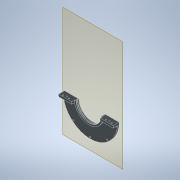
# Autodesk Inventor part: Крышка стенки картера низ
Saved by Autodesk Inventor 2021 (Build 250183000, 183)
## iProperties
Created: 2020-12-05
Part Number: Крышка стенки картера низ
Material: Чугун, серый
Document SubType Name: Modeling
Designer: Тимоха
Density: 7.15 g/cm^3
Appearance: Чугун серый
Mass: 3617.17 g
Surface Area: 1231.32 cm^2
Volume: 505.898 cm^3
Author: Тимоха
Autodesk Inventor part; units mm, degrees
ref_plane "YZ Plane" through (0, 0, 0) normal (1, 0, 0) x (0, 1, 0)
ref_plane "XZ Plane" through (0, 0, 0) normal (0, 1, 0) x (-1, 0, 0)
ref_plane "XY Plane" through (0, 0, 0) normal (0, 0, 1) x (1, 0, 0)
ref_plane "РабПлоскость1" through (7.7596, 35.7122, 0) normal (0, 0, 1) x (1, 0, 0)
sketch "Эскиз1" plane through (7.7596, 35.7122, 0) normal (0, 0, 1) x (1, 0, 0)
  circle A0 centre (-7.7596, -110.7122) radius 100 projected
  line L0 (177.2404, -110.7122) -> (177.2404, 289.2878) projected
  line L1 (157.2404, 304.2878) -> (157.2404, -110.7122) projected
  arc A1 (-172.7596, -110.7122) -> (157.2404, -110.7122) centre (-7.7596, -110.7122) ccw projected
  line L2 (-172.7596, -110.7122) -> (-172.7596, 304.2878) projected
  line L3 (-192.7596, 289.2878) -> (-192.7596, -110.7122) projected
  arc A2 (-192.7596, -110.7122) -> (177.2404, -110.7122) centre (-7.7596, -110.7122) ccw projected
  line L4 (-192.7596, -110.7122) -> (177.2404, -110.7122)
  circle A3 centre (-7.7596, -110.7122) radius 86
  line L5 (177.2404, 289.2878) -> (222.2404, 289.2878) projected
  line L6 (222.2404, 289.2878) -> (222.2404, 304.2878) projected
  line L7 (222.2404, 304.2878) -> (157.2404, 304.2878) projected
  line L8 (-172.7596, 304.2878) -> (-237.7596, 304.2878) projected
  line L9 (-237.7596, 304.2878) -> (-237.7596, 289.2878) projected
  line L10 (-237.7596, 289.2878) -> (-192.7596, 289.2878) projected
  point P0 (-7.7596, -35.7122)
  point P1 (177.2404, 304.2878)
  point P2 (-192.7596, 304.2878)
  point P3 (157.2404, -110.7122)
  point P4 (78.2404, -110.7122)
  point P5 (-93.7596, -110.7122)
  point P6 (-172.7596, -110.7122)
  dimension "d2" = 172
  constraints: 2 end point, 2 point on line, 1 centre point, 1 coincident, 1 perpendicular
  measures "d2" diameter of A3
extrude "Выдавливание1" add sketch "Эскиз1" along normal blind 10 contours L4 A1 A0 | A0 L4 A3 | L4 A2 A1 picked at (-5.6173, -205.81)
sketch "Эскиз2" plane through (7.7596, 35.7122, 10) normal (0, 0, 1) x (1, 0, 0)
  arc A0 (-93.7596, -110.7122) -> (78.2404, -110.7122) centre (-7.7596, -110.7122) ccw projected
  line L0 (-93.7596, -110.7122) -> (78.2404, -110.7122) projected
  line L1 (-93.7596, -110.7122) -> (78.2404, -110.7122) projected
  circle A1 centre (-7.7596, -110.7122) radius 97.5
  line L2 (-93.7596, -110.7122) -> (-105.2596, -110.7122)
  line L3 (78.2404, -110.7122) -> (89.7404, -110.7122)
  point P0 (-7.7596, -35.7122)
  point P1 (-172.7596, -110.7122)
  point P2 (157.2404, -110.7122)
  point P3 (-105.2596, -110.7122)
  point P4 (89.7404, -110.7122)
  point P5 (177.2404, -110.7122)
  dimension "d3" = 195
  constraints: 4 end point, 2 point on circle, 1 centre point, 1 coincident, 1 point on line
  measures "d3" diameter of A1
extrude "Выдавливание2" add sketch "Эскиз2" along normal blind 10 contours A0 L3 A1 L2
sketch "Эскиз3" plane through (0, 0, 0) normal (1, 0, 0) x (0, 1, 0)
  line L0 (-161, 20) -> (-75, 20) projected
  line L1 (-161, 20) -> (-161, 17)
  line L2 (-161, 20) -> (-161, 0) projected
  line L3 (-161, 17) -> (-168, 17)
  line L4 (-168, 17) -> (-168, 12)
  line L5 (-168, 12) -> (-161, 12)
  line L6 (-161, 12) -> (-161, 9)
  line L7 (-161, 9) -> (-168, 9)
  line L8 (-168, 9) -> (-168, 3)
  line L9 (-168, 3) -> (-161, 3)
  line L10 (-161, 0) -> (-75, 0) projected
  line L11 (-161, 3) -> (-161, 0)
  line L12 (-161, 0) -> (-168, 0)
  line L13 (-75, 0) -> (-75, 20) projected
  point P0 (0, 0)
  point P1 (-75, 10)
  constraints: 20 end point, 7 point on line, 5 perpendicular, 1 horizontal
revolve "Вращение1" cut sketch "Эскиз3" angle 360 about axis through (0, -75, 0) along (0, 0, 1) contours L2 L5 L4 L3 | L2 L9 L8 L7
sketch "Эскиз4" plane through (7.7596, 35.7122, 10) normal (0, 0, 1) x (1, 0, 0)
  arc A0 (-105.2596, -110.7122) -> (89.7404, -110.7122) centre (-7.7596, -110.7122) ccw projected
  line L0 (-105.2596, -110.7122) -> (-192.7596, -110.7122) projected
  line L1 (177.2404, -110.7122) -> (89.7404, -110.7122) projected
  line L2 (-105.2596, -110.7122) -> (-192.7596, -110.7122) projected
  arc A1 (-105.2596, -110.7122) -> (89.7404, -110.7122) centre (-7.7596, -110.7122) ccw projected
  line L3 (177.2404, -110.7122) -> (78.2404, -110.7122) projected
  arc A2 (-192.7596, -110.7122) -> (177.2404, -110.7122) centre (-7.7596, -110.7122) ccw projected
  line L4 (-192.7596, -110.7122) -> (-192.7596, -125.7122)
  line L5 (-192.7596, -125.7122) -> (-104.0989, -125.7122)
  line L6 (177.2404, -110.7122) -> (177.2404, -125.7122)
  line L7 (177.2404, -110.7122) -> (177.2404, -110.7122) projected
  line L8 (177.2404, -125.7122) -> (88.5796, -125.7122)
  point P0 (-7.7596, -35.7122)
  point P1 (-104.0989, -125.7122)
  point P2 (88.5796, -125.7122)
  point P3 (176.6313, -125.7122)
  point P4 (-192.1505, -125.7122)
  dimension "d23" = 15
  constraints: 8 end point, 3 point on line, 2 point on circle, 1 perpendicular
  measures "d23" distance of L0.end L4.end
extrude "Выдавливание3" add sketch "Эскиз4" along normal blind 30 contours A0 L5 A2 L0 | A0 L1 A2 L8
sketch "Эскиз5" plane through (86, -75, 0) normal (0, 1, 0) x (1, 0, 0)
  line L0 (-86, 0) -> (-86, -49)
  line L1 (-271, 0) -> (-271, -40) projected
  line L2 (-271, -40) -> (-271, -30)
  line L3 (-271, -30) -> (-251, -30)
  line L4 (-251, -30) -> (-211, -30)
  point P0 (79, -30)
  point P1 (39, -30)
  point P2 (-271, -10)
  dimension "d24" = 10
  constraints: 8 end point, 2 point on line, 2 symmetric about line, 1 perpendicular, 1 vertical
  measures "d24" distance of L1.end L2.end
hole "Отверстие1" at (-165, -75, 30) at (-125, -75, 30) at (125, -75, 30) at (165, -75, 30) direction (0, -1, 0) diameter 8 end through all
sketch "Эскиз7" plane through (-185, -75, 0) normal (0, 1, 0) x (1, 0, 0)
  line L0 (185, 0) -> (185, -43)
  point P0 (41, -24)
  point P1 (329, -24)
  constraints: 2 end point, 1 symmetric about line, 1 vertical
hole "Отверстие3" at (-144, -75, 24) at (144, -75, 24) direction (0, -1, 0) diameter 6 end through all
sketch "Эскиз8" plane through (7.7596, 35.7122, 10) normal (0, 0, 1) x (1, 0, 0)
  arc A0 (-192.7596, -110.7122) -> (177.2404, -110.7122) centre (-7.7596, -110.7122) ccw projected
  arc A1 (-180.8984, -136.1673) -> (165.3791, -136.1673) centre (-7.7596, -110.7122) ccw
  point P0 (-7.7596, -35.7122)
  point P1 (-192.1505, -125.7122)
  point P2 (176.6313, -125.7122)
  dimension "d43" = 10
  constraints: 2 point on circle, 1 centre point
  measures "d43" radial gap between concentric circles of A0 A1
hole "Отверстие4" at (-173.1388, -100.4552, 10) direction (0, 0, -1) diameter 9 end through all
pattern_circular "Круговой массив1" count 5 over 163 about axis through (0, -75, 10) along (0, 0, 1) of "Отверстие4"
